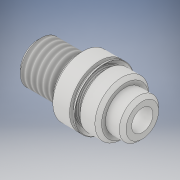
# Autodesk Inventor part: 007000-0_rod_guide
Saved by Autodesk Inventor 2018 (Build 220112000, 112)
## iProperties
Created: 2019-01-16
Part Number: 007000-0_rod_guide
Material: Generic
Catalog Web Link: www.cadenas.de
Description: Rod Guide-Original Line - Standard Air Cylinders
Vendor: BIMBA
Document SubType Name: Modeling
Designer: s-4008082
Manufacturer: BIMBA
Mass: 0.526118 g
Surface Area: 6.64661 cm^2
Volume: 0.526118 cm^3
Density: 1 g/cm^3
Appearance: PSOLRGB-211-211-211
Category: PARTsolutions
Company: BIMBA
Title: 007000-0_rod_guide
Author: Cadenas PARTsolutions
Comments: Original Line - Standard Air Cylinders
PSOL_IDENT_0: {$CADENAS_DATA\23d-libs\bimba\bimba\bimba_imperial\bimba_full_line\original_line_cylinders\standard_
PSOL_IDENT_1: air_cylinders\rod_guide.prj},251 {VTYP=3D},{NB=007000-0_rod_guide},{LINA=007000-0_rod_guide},{NN=Rod
PSOL_IDENT_2: Guide},{DATE=21.03.2018 14:31:21},{GEOMDATE=09.11.2017 12:44:00},{VERSION=},{LINEID=10},{WBVAR=MNT,
PSOL_IDENT_3: ACTING,NR,K,Q,T1,T2,T3,T4,MB,TRIM,CUSH,RODTRANS},{WBNUMERIC=MB,TRIM,CUSH,RODTRANS}  {NB=007000-0_rod
PSOL_IDENT_4: _guide},{LINA=007000-0_rod_guide},{KT=DUMMY},{PN=007000},{BORE=0.31250000},{BOREPN=007},{MNT=},{MNTA
PSOL_IDENT_5: LG='' , 'Front Nose' , 'BF' , 'Front Block'},{ACTING=},{ACTINGALG= '' , 'Single Acting' , 'R' , 'Rev
PSOL_IDENT_6: erse/Double Acting' },{NR=},{NRALG= '' , 'N/A' },{K=},{Q=},{QALG= '' , 'Without Side Ported Rear Hea
PSOL_IDENT_7: d' , 'Q' , 'With Side Ported Rear Head' },{T1=},{T2=},{T3=},{T4=},{MB=0},{A1=0.6250},{A1N=0.6250},{A
PSOL_IDENT_8: 1P=0.8450},{A1B=0.9060},{A2=0.2500},{A2N=0.2500},{A2P=0.3120},{A3=0.1200},{A3N=0.1200},{A3P=0.3125},
PSOL_IDENT_9: {A4=0.2550},{A4N=0.2550},{A4P=0.1585},{A5=0.0220},{A6=0.1025},{A6N=0.1025},{A6P=0.0000},{A7=0.2050},
PSOL_IDENT_10: {A7N=0.2050},{A7P=0.3040},{A8=0.0150},{A8N=0.0150},{A8NR=0.0150},{D1=0.3590},{D1N=0.3590},{D1P=0.605
PSOL_IDENT_11: 0},{D1B=0.0000},{D2=0.3215},{D3=0.2350},{D3N=0.2350},{D3P=0.0000},{D4=0.1420},{D4N=0.1420},{D4P=0.15
PSOL_IDENT_12: 30},{D4NR=0.1530},{D5=0.1280},{D5N=0.1280},{D5NR=0.1280},{C1=0.020},{C2=0.0200},{C2N=0.0200},{C2P=0.
PSOL_IDENT_13: 0200},{C3=0.0000},{C3N=0.0000},{C3P=0.0300},{C4=0.0200},{C4N=0.0200},{C4P=0.0300},{NDM=0.2500},{NDMN=
PSOL_IDENT_14: 0.2500},{NDMP=0.3750},{TAB=UNF},{D6=0.0000},{D6N=0.0000},{D6P=0.0000},{A9=0.0000},{A9N=0.0000},{A9P=
PSOL_IDENT_15: 0.0000},{D7=0.0000},{D7N=0.0000},{D7P=0.0000},{A10=0.0000},{A10N=0.0000},{A10P=0.0000},{R1=0.0000},{
PSOL_IDENT_16: R1N=0.0000},{R1P=0.0000},{D8=0.0000},{D9=0.0000},{D10=0.0000},{A11=0.0000},{A12=0.0000},{A13=0.0000}
PSOL_IDENT_17: ,{A14=0.3750},{A14N=0.3750},{A14B=0.5000},{D11=0.0000},{D11N=0.0000},{NDM2=0.1900},{NDM2N=0.1900},{N
PSOL_IDENT_18: DM2DP=0.0000},{THREAD=1},{HEX=0.0000},{HEXN=0.0000},{S1=0.5000},{B1=0.0620},{B2=0.5940},{B22=0.0000}
PSOL_IDENT_19: ,{DB=0.1130},{B3=0.0150},{B4=0.3430},{X1=0.0000},{X2=0.0000},{NDM3=0.0000},{NDM4=0.0000},{NDM4DP=0.0
PSOL_IDENT_20: 000},{DD=0.0000},{CB=0.0000},{CBDP=0.0000},{PORT=1},{XT=0.0000},{XTX=0.0000},{XT1=0.0000},{XT2=0.000
PSOL_IDENT_21: 0},{NDMH=0.0000},{OD=0.3590},{ID=0.3215},{G=0.0000},{PNUT=0.2500},{TRIM=0},{C11=0.0000},{C22=0.0000}
PSOL_IDENT_22: ,{C33=0.0000},{C44=0.0000},{C55=0.0000},{CD1=0.0000},{CD2=0.0000},{CD3=0.0000},{CNDM3=0.0000},{CTAB3=
PSOL_IDENT_23: 0.0000},{CUSH=0},{XX=0.34300},{LCD=0.0000},{RODTRANS=0.00000}
NN: Rod Guide
NT: Original Line - Standard Air Cylinders
NB: 007000-0_rod_guide
NBSYN: $PN.-$RODTRANS._rod_guide
LINA: 007000-0_rod_guide
BORE: 0
BOREPN: 007
MNT: Front Nose
MNTALG: '' , 'Front Nose' , 'BF' , 'Front Block'
ACTING: Single Acting
NR: N/A
K: Standard
Q: Without Side Ported Rear Head
T1: without T1
T2: without T2
T3: without T3
T4: without T4
MB: 0
A1N: 0.625
A1P: 0.845
A1B: 0.906
A2N: 0.25
A2P: 0.312
A3N: 0.12
A3P: 0.3125
A4N: 0.255
A4P: 0.1585
A5: 0.022
A6N: 0.1025
A6P: 0
A7N: 0.205
A7P: 0.304
A8N: 0.015
A8NR: 0.015
D1N: 0.359
D1P: 0.605
D1B: 0
D2: 0.3215
D3N: 0.235
D3P: 0
D4N: 0.142
D4P: 0.153
D4NR: 0.153
D5N: 0.128
D5NR: 0.128
C1: 0.02
C2N: 0.02
C2P: 0.02
C3N: 0
C3P: 0.03
C4N: 0.02
C4P: 0.03
NDMN: 0.25
NDMP: 0.375
TAB: UNF
D6N: 0
D6P: 0
A9N: 0
A9P: 0
D7N: 0
D7P: 0
A10N: 0
A10P: 0
R1N: 0
R1P: 0
D8: 0
D9: 0
D10: 0
A11: 0
A12: 0
A13: 0
A14N: 0.375
A14B: 0.5
D11N: 0
NDM2N: 0.19
NDM2DP: 0
HEXN: 0
S1: 0.5
B1: 0.062
B2: 0.594
B22: 0
DB: 0.113
B3: 0.015
B4: 0.343
X1: 0
X2: 0
NDM3: 0
NDM4: 0
NDM4DP: 0
DD: 0
CB: 0
CBDP: 0
XTX: 0
XT1: 0
XT2: 0
NDMH: 0
TRIM: 0
C11: 0
C22: 0
C33: 0
C44: 0
C55: 0
CD1: 0
CD2: 0
CD3: 0
CNDM3: 0
CTAB3: 0.0000
CUSH: 0
LCD: 0
RODTRANS: 0
SUPPLIER: BIMBA
ARTICLENO: 007000-0_rod_guide
BOMINFO: 007000-0_rod_guide
CREATOR: CADENAS GmbH
Autodesk Inventor part; units mm, degrees
sketch "Sketch_1" plane through (0, 0, 0) normal (0, 0, 1) x (1, 0, 0)
  line L0 (6.35, 0) -> (0, 0)
  line L1 (0, 0) -> (0, 2.634)
  line L2 (0, 2.634) -> (0.541, 3.175)
  line L3 (0.541, 3.175) -> (6.35, 3.175)
  line L4 (6.35, 3.175) -> (6.35, 0)
  line L5 (6.35, 0) -> (0, 0)
  constraints: 12 end point
revolve "Revolution1" add sketch "Sketch_1" angle 360 about axis through (6.35, 0, 0) along (1, 0, 0)
thread "Thread1" size "1/4-28 UNF" class "2A" standard "ANSI Unified Screw Threads" full length
sketch "Sketch_3" plane through (0, 0, 0) normal (0, 0, 1) x (1, 0, 0)
  line L0 (13.2715, 0) -> (6.35, 0)
  line L1 (6.35, 0) -> (6.35, 4.0513)
  line L2 (6.35, 4.0513) -> (6.858, 4.5593)
  line L3 (6.858, 4.5593) -> (9.398, 4.5593)
  line L4 (9.398, 4.5593) -> (9.398, 3.5242)
  line L5 (9.398, 3.5242) -> (9.9568, 3.5242)
  line L6 (9.9568, 3.5242) -> (10.5156, 4.0831)
  line L7 (10.5156, 4.0831) -> (12.7635, 4.0831)
  line L8 (12.7635, 4.0831) -> (13.2715, 3.5751)
  line L9 (13.2715, 3.5751) -> (13.2715, 0)
  line L10 (13.2715, 0) -> (6.35, 0)
  constraints: 22 end point
revolve "Revolution2" add sketch "Sketch_3" angle 360 about axis through (13.2715, 0, 0) along (1, 0, 0)
sketch "Sketch_4" plane through (0, 0, 0) normal (0, 0, 1) x (1, 0, 0)
  line L0 (15.875, 0) -> (13.2715, 0)
  line L1 (13.2715, 0) -> (13.2715, 2.9845)
  line L2 (13.2715, 2.9845) -> (15.367, 2.9845)
  line L3 (15.367, 2.9845) -> (15.875, 2.4765)
  line L4 (15.875, 2.4765) -> (15.875, 0)
  line L5 (15.875, 0) -> (13.2715, 0)
  constraints: 12 end point
revolve "Revolution3" add sketch "Sketch_4" angle 360 about axis through (15.875, 0, 0) along (1, 0, 0)
sketch "Sketch4" plane through (0, 0, 0) normal (-1, 0, 0) x (0, 0, 1)
  point P0 (0, 0)
hole "Hole1" at (0, 0, 0) direction (1, 0, 0) diameter 3.2512 depth 15.875 countersink diameter 4.0132 countersink angle 90
sketch "Sketch_47" plane through (0, 0, 0) normal (0, 0, 1) x (1, 0, 0)
  line L0 (9.9568, 0) -> (9.398, 0)
  line L1 (9.398, 4.0431) -> (9.398, 3.2702)
  line L2 (9.398, 3.2702) -> (9.9568, 3.2702)
  line L3 (9.9568, 3.2702) -> (9.9568, 3.5242)
  line L4 (9.9568, 3.5242) -> (9.6774, 3.5242)
  line L5 (9.6774, 3.5242) -> (9.5118, 3.6899)
  arc A0 (9.5118, 3.8695) -> (9.5118, 3.6899) centre (9.6016, 3.7797) ccw
  line L6 (9.5118, 3.8695) -> (10.1174, 4.4751)
  line L7 (10.1174, 4.4751) -> (10.1174, 4.5593)
  line L8 (10.1174, 4.5593) -> (9.9142, 4.5593)
  line L9 (9.9142, 4.5593) -> (9.398, 4.0431)
  constraints: 20 end point, 2 point on circle, 1 centre point
revolve "Revolution4" add sketch "Sketch_47" angle 360 about axis through (9.9568, 0, 0) along (1, 0, 0)
ref_plane "hh_XY" through (0, 3.175, 0) normal (0, 0, 1) x (1, 0, 0)
ref_plane "hh_YZ" through (0, 3.175, 0) normal (1, 0, 0) x (0, 1, 0)
ref_plane "hh_ZX" through (0, 3.175, 0) normal (0, 1, 0) x (0, 0, 1)
ref_plane "rod_guide_XY" through (0, 0, 0) normal (1, 0, 0) x (0, 0, -1)
ref_plane "rod_guide_YZ" through (0, 0, 0) normal (0, 0, -1) x (0, 1, 0)
ref_plane "rod_guide_ZX" through (0, 0, 0) normal (0, 1, 0) x (1, 0, 0)
ref_plane "t1_XY" through (6.35, 0, 0) normal (1, 0, 0) x (0, 0, -1)
ref_plane "t1_YZ" through (6.35, 0, 0) normal (0, 0, -1) x (0, 1, 0)
ref_plane "t1_ZX" through (6.35, 0, 0) normal (0, 1, 0) x (1, 0, 0)
ref_plane "t111_XY" through (6.35, 0, 0) normal (1, 0, 0) x (0, 0, -1)
ref_plane "t111_YZ" through (6.35, 0, 0) normal (0, 0, -1) x (0, 1, 0)
ref_plane "t111_ZX" through (6.35, 0, 0) normal (0, 1, 0) x (1, 0, 0)
ref_plane "to_foot_bracket_XY" through (6.35, 0, 0) normal (1, 0, 0) x (0, 0, -1)
ref_plane "to_foot_bracket_YZ" through (6.35, 0, 0) normal (0, 0, -1) x (0, 1, 0)
ref_plane "to_foot_bracket_ZX" through (6.35, 0, 0) normal (0, 1, 0) x (1, 0, 0)
ref_plane "to_nut_XY" through (6.35, 0, 0) normal (1, 0, 0) x (0, 0, -1)
ref_plane "to_nut_YZ" through (6.35, 0, 0) normal (0, 0, -1) x (0, 1, 0)
ref_plane "to_nut_ZX" through (6.35, 0, 0) normal (0, 1, 0) x (1, 0, 0)
ref_plane "to_rod_XY" through (0, 0, 0) normal (1, 0, 0) x (0, 0, -1)
ref_plane "to_rod_YZ" through (0, 0, 0) normal (0, 0, -1) x (0, 1, 0)
ref_plane "to_rod_ZX" through (0, 0, 0) normal (0, 1, 0) x (1, 0, 0)
ref_plane "to_screw_XY" through (6.35, 0, 0) normal (0, 1, 0) x (1, 0, 0)
ref_plane "to_screw_YZ" through (6.35, 0, 0) normal (1, 0, 0) x (0, 0, -1)
ref_plane "to_screw_ZX" through (6.35, 0, 0) normal (0, 0, -1) x (0, 1, 0)
ref_plane "to_trunnion_brackets_XY" through (0, 0, 0) normal (0, 1, 0) x (1, 0, 0)
ref_plane "to_trunnion_brackets_YZ" through (0, 0, 0) normal (1, 0, 0) x (0, 0, -1)
ref_plane "to_trunnion_brackets_ZX" through (0, 0, 0) normal (0, 0, -1) x (0, 1, 0)
ref_plane "to_trunnion_brackets1_XY" through (0, 6.35, 0) normal (0, 1, 0) x (1, 0, 0)
ref_plane "to_trunnion_brackets1_YZ" through (0, 6.35, 0) normal (1, 0, 0) x (0, 0, -1)
ref_plane "to_trunnion_brackets1_ZX" through (0, 6.35, 0) normal (0, 0, -1) x (0, 1, 0)
ref_plane "to_trunnion_brackets2_XY" through (0, -6.35, 0) normal (0, 1, 0) x (1, 0, 0)
ref_plane "to_trunnion_brackets2_YZ" through (0, -6.35, 0) normal (1, 0, 0) x (0, 0, -1)
ref_plane "to_trunnion_brackets2_ZX" through (0, -6.35, 0) normal (0, 0, -1) x (0, 1, 0)
ref_plane "to_tube_XY" through (9.9568, 0, 0) normal (1, 0, 0) x (0, 0, -1)
ref_plane "to_tube_YZ" through (9.9568, 0, 0) normal (0, 0, -1) x (0, 1, 0)
ref_plane "to_tube_ZX" through (9.9568, 0, 0) normal (0, 1, 0) x (1, 0, 0)
body "Solid1"
